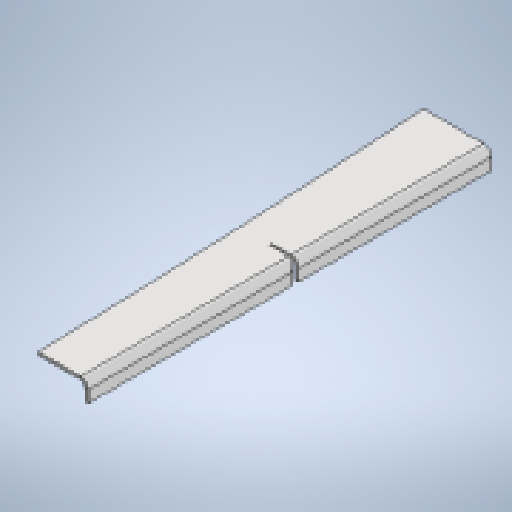
# Autodesk Inventor part: MSC 348 RIB BOARD
Saved by Autodesk Inventor 2025.1 (Build 291241020, 241B)
## iProperties
Created: 2024-04-28
Part Number: MSC 348 RIB BOARD
Material: Stainless Steel
Description: DIE16(5)|\ 90°|corrY -___°|X_____|bom___
Document SubType Name: Sheet Metal
Designer: user
Stock Number: МОО 340 шпангоут борт
Mass: 1762.25 g
Surface Area: 2283.33 cm^2
Volume: 220.281 cm^3
Density: 8 g/cm^3
Flat Pattern Width: 8.39274 cm
Flat Pattern Length: 52 cm
Flat Pattern Area: 436.423 cm^2
Sheet Metal Rule: AISI304 3mm Die 32
Sheet Metal Width: 83.927 mm
Sheet Metal Length: 520.000 mm
Sheet Metal Area: 43642.265 mm^2
Appearance: Default
Author: admin
БОРТ_стрингер_3_высота: 59.000 mm
БОРТ_стрингер_4_высота: 48.000 mm
БОРТ_стрингер_5_высота: 53.000 mm
БОРТ_стрингер_6_высота: 72.000 mm
РЕБРА_глубина_паза: 28.000 mm
РЕБРА_вырез_на_полке: 5,000 mm
РЕБРА_полка: 20,000 mm
Autodesk Inventor part; units mm, degrees
ref_plane "YZ Plane" through (0, 0, 0) normal (1, 0, 0) x (0, 1, 0)
ref_plane "XZ Plane" through (0, 0, 0) normal (0, 1, 0) x (-1, 0, 0)
ref_plane "XY Plane" through (0, 0, 0) normal (0, 0, 1) x (1, 0, 0)
sketch "Sketch1" plane through (0, 0, 0) normal (0, 0, 1) x (1, 0, 0)
  arc A0 (-97, -1740) -> (-70, 0) centre (-11100.8726, -699.0408) ccw
  line L0 (0, 0) -> (-70, 0)
  line L1 (0, -16.732) -> (-68.9524, -16.732) construction
  line L2 (0, -496.732) -> (-49.7243, -496.732) construction
  line L3 (0, -976.732) -> (-51.3615, -976.732) construction
  line L4 (0, -1456.732) -> (-73.8734, -1456.732) construction
  line L5 (-97, -1740) -> (0, -1740)
  line L6 (0, 0) -> (0, -1740)
  line L7 (0, -1730) -> (-10.3553, -1740)
  point P0 (-20, 0)
  dimension "d33" = 50
  dimension "d58" = 480
  dimension "d59" = 480
  dimension "d60" = 480
  dimension "d141" = 1740
  dimension "d148" = 70
  dimension "d149" = 11053
  dimension "d150" = 97
  dimension "d151" = 136
  dimension "d153" = 10
  measures "d33" distance of L0.end point (-20, 0)
  measures "d58" distance between parallel lines of L2 L1
  measures "d59" distance between parallel lines of L2 L3
  measures "d60" distance between parallel lines of L3 L4
  measures "d141" distance between parallel lines of L0 L5
  measures "d148" distance of L0.start L0.end
  measures "d149" radius of A0
  measures "d150" distance of L5.start L5.end
  measures "d151" angle of L5 L7
  measures "d153" distance of L5.end L7.start
extrude "Plate3" add sketch "Sketch1" along normal blind 3 contours A0 L0 L6 L7 L5
sketch "Sketch3" plane through (-3, 0, 3) normal (1, 0, 0) x (0, 1, 0)
  line L0 (-1730, 0) -> (0, 0)
  line L1 (0, 0) -> (0, 20)
  line L2 (0, 20) -> (-1730, 20)
  line L3 (-1730, 20) -> (-1730, 0)
  constraints: 6 end point, 1 horizontal, 1 perpendicular, 1 vertical
edge flange "Flange2" height 20 angle 90 thickness 3 bend radius 5 thickness toward (1, 0, 0) relief round relief width 3 relief depth 1.5 edges at (0, -865, 3) wall of the first edge with corners at (-3, -1730, 3) (-3, 0, 3) (-3, 0, -17) (-3, -1730, -17)
bend "Bend2"
corner "Corner2"
sketch "Sketch5" plane through (0, 0, 0) normal (0, 0, 1) x (1, 0, 0)
  line L0 (-8, -1737.7255) -> (-8, 0) projected
  line L1 (-70, 0) -> (-8, 0) projected
  arc A0 (-97, -1740) -> (-70, 0) centre (-11100.8726, -699.0408) ccw projected
  line L2 (0, 0) -> (0, -1730) projected
  line L3 (0, -198.9) -> (-28, -198.9)
  line L4 (0, -201.1) -> (-3, -201.1)
  line L5 (-3, -1730) -> (-3, 0) projected
  line L6 (-28, -198.9) -> (-28, -201.1)
  line L7 (0, -608.9) -> (-48.2402, -608.9) construction
  line L8 (0, -1018.9) -> (-52.5018, -1018.9) construction
  line L9 (0, -1428.9) -> (-71.9962, -1428.9) construction
  line L10 (-10.3553, -1740) -> (-97, -1740) projected
  line L11 (0, -198.9) -> (0, -218.9)
  line L12 (-3, -198.9) -> (-3, -201.1) construction
  line L13 (0, -218.9) -> (-3, -218.9)
  line L14 (-28, -198.9) -> (-59.1939, -198.9) construction
  line L15 (-28, -201.1) -> (-59.0945, -201.1) construction
  line L16 (-3, -201.1) -> (-3, -218.9)
  line L17 (-3, -201.1) -> (-28, -201.1)
  line L18 (-3, -218.9) -> (-8, -218.9)
  line L19 (-8, -1737.7255) -> (-10.3553, -1740) projected
  line L20 (-4.4351, -201.1) -> (0, -205.5351)
  line L21 (-4.4351, -201.1) -> (1.8371, -201.1) construction
  line L22 (-10.3553, -1740) -> (-10.3553, -1770)
  point P0 (0, 0)
  point P1 (845.25, -380.4205)
  point P2 (848, -380.4205)
  point P3 (-28, -200)
  point P4 (850, -410.4205)
  point P5 (-3, -198.9)
  point P6 (-3, -218.9)
  point P7 (-8, -201.1)
  point P8 (0, -205.5351)
  dimension "d69" = 1730
  dimension "d70" = 2.2
  dimension "d76" = 59.1939
  dimension "d80" = 48.2402
  dimension "d102" = 71.9962
  dimension "d104" = 52.5018
  dimension "d106" = 3
  dimension "d107" = 20
  dimension "d108" = 200
  dimension "d112" = 28
  dimension "d142" = 410
  dimension "d143" = 410
  dimension "d144" = 410
  dimension "d154" = 45
  dimension "d155" = 30
  dimension "d156" = 341.1
  constraints: 34 end point, 13 perpendicular, 12 point on line, 5 point on circle, 2 horizontal, 2 parallel, 1 equal length, 1 midpoint, 1 vertical
  measures "d69" distance of L2.start L2.end
  measures "d70" distance between parallel lines of L4 L3
  measures "d76" distance of L3.start L14.end
  measures "d80" distance of L7.start L7.end
  measures "d102" distance of L9.start L9.end
  measures "d104" distance of L8.end L8.start
  measures "d106" distance of L13.end L11.end
  measures "d107" distance of L11.end L3.start
  measures "d108" vertical distance of L2.start point (-28, -200)
  measures "d112" distance of L3.end L3.start
  measures "d142" distance between parallel lines of L7 L14
  measures "d143" distance between parallel lines of L7 L8
  measures "d144" distance between parallel lines of L9 L8
  measures "d154" angle of L20 L21
  measures "d155" distance of L10.start L22.end
  measures "d156" distance from line of L9 L22.end
extrude "Extrusion2" cut sketch "Sketch5" along normal through all both and the other way through all contours L17 L6 L3 L0 | L0 L3 L5 L17 | L17 L5 L20 | L5 L4 L2 L20 | L3 L2 L4 L5
pattern_linear "Rectangular Pattern3" count 4 spacing 410 along (0, -1, 0) of "Extrusion2"
sketch "Sketch7" plane through (0, 0, 0) normal (0, 0, 1) x (1, 0, 0)
  line L0 (0, 0) -> (0, -198.9) projected
  line L1 (0, 0) -> (-100, 0)
  line L2 (-100, 0) -> (-100, -520)
  line L3 (-100, -520) -> (0, -520)
  line L4 (0, -520) -> (0, 0)
  line L5 (-100, -1740) -> (0, -1740)
  line L6 (0, -1740) -> (0, -520)
  line L7 (0, -520) -> (-100, -520)
  line L8 (-100, -520) -> (-100, -1740)
  line L9 (-97, -1740) -> (-10.3553, -1740) projected
  point P0 (-50, -1740)
  dimension "d157" = 100
  dimension "d158" = 520
  constraints: 16 end point, 4 parallel, 2 horizontal, 2 perpendicular, 1 midpoint, 1 point on line
  measures "d157" distance of L3.end L2.end
  measures "d158" distance of L2.end L1.end
extrude "Extrusion3" cut sketch "Sketch7" along normal through all both and the other way through all contours L6 L5 L8 L3
equation "\"d33\" = d25"
equation "\"БОРТ_стрингер_3_высота\" = 59"
equation "\"БОРТ_стрингер_4_высота\" = 48"
equation "\"БОРТ_стрингер_5_высота\" = 53"
equation "\"БОРТ_стрингер_6_высота\" = 72"
equation "\"d25\" = 50"
body "Solid2"
